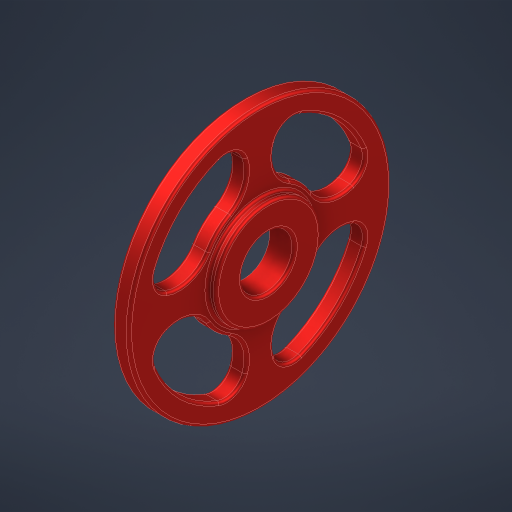
# Autodesk Inventor part: Part5
Saved by Autodesk Inventor 2024 (Build 280153000, 153)
## iProperties
Created: 2024-03-07
Part Number: Part5
Material: Aluminum, Anodized Red
Document SubType Name: Modeling
Designer: Papryk
Density: 2.7 g/cm^3
Appearance: Anodized - Red
Author: Papryk
Autodesk Inventor part; units mm, degrees
ref_plane "YZ Plane" through (0, 0, 0) normal (1, 0, 0) x (0, 1, 0)
ref_plane "XZ Plane" through (0, 0, 0) normal (0, 1, 0) x (-1, 0, 0)
ref_plane "XY Plane" through (0, 0, 0) normal (0, 0, 1) x (1, 0, 0)
sketch "Sketch1" plane through (0, 0, 0) normal (1, 0, 0) x (0, 1, 0)
  arc A0 (15.3115, -37.4941) -> (37.7556, -14.6548) centre (0, 0) ccw
  arc A1 (11.2212, -18.9232) -> (19.1161, -10.8892) centre (0, 0) ccw
  arc A2 (33.5916, -5.5323) -> (19.1161, -10.8892) centre (29.5431, -16.8287) ccw
  arc A3 (11.2212, -18.9232) -> (6.1177, -33.4899) centre (17.3418, -29.2449) ccw
  arc A4 (37.7556, -14.6548) -> (33.5916, -5.5323) centre (31.2299, -12.1219) ccw
  arc A5 (6.1177, -33.4899) -> (15.3115, -37.4941) centre (12.6651, -31.0136) ccw
  arc A6 (0, -47.5) -> (47.5, 0) centre (0, 0) ccw
  arc A7 (0, -19) -> (19, 0) centre (0, 0) ccw
  arc A8 (0, -9.5) -> (9.5, 0) centre (0, 0) ccw
  arc A9 (-37.7556, -14.6548) -> (-15.3115, -37.4941) centre (0, 0) ccw
  arc A10 (-19.1161, -10.8892) -> (-11.2212, -18.9232) centre (0, 0) ccw
  arc A11 (-19.1161, -10.8892) -> (-33.5916, -5.5323) centre (-29.5431, -16.8287) ccw
  arc A12 (-6.1177, -33.4899) -> (-11.2212, -18.9232) centre (-17.3418, -29.2449) ccw
  arc A13 (-33.5916, -5.5323) -> (-37.7556, -14.6548) centre (-31.2299, -12.1219) ccw
  arc A14 (-15.3115, -37.4941) -> (-6.1177, -33.4899) centre (-12.6651, -31.0136) ccw
  arc A15 (-47.5, 0) -> (0, -47.5) centre (0, 0) ccw
  arc A16 (-19, 0) -> (0, -19) centre (0, 0) ccw
  arc A17 (-9.5, 0) -> (0, -9.5) centre (0, 0) ccw
  arc A18 (37.7556, 14.6548) -> (15.3115, 37.4941) centre (0, 0) ccw
  arc A19 (19.1161, 10.8892) -> (11.2212, 18.9232) centre (0, 0) ccw
  arc A20 (19.1161, 10.8892) -> (33.5916, 5.5323) centre (29.5431, 16.8287) ccw
  arc A21 (6.1177, 33.4899) -> (11.2212, 18.9232) centre (17.3418, 29.2449) ccw
  arc A22 (33.5916, 5.5323) -> (37.7556, 14.6548) centre (31.2299, 12.1219) ccw
  arc A23 (15.3115, 37.4941) -> (6.1177, 33.4899) centre (12.6651, 31.0136) ccw
  arc A24 (47.5, 0) -> (0, 47.5) centre (0, 0) ccw
  arc A25 (19, 0) -> (0, 19) centre (0, 0) ccw
  arc A26 (9.5, 0) -> (0, 9.5) centre (0, 0) ccw
  arc A27 (-37.7556, 14.6548) -> (-33.5916, 5.5323) centre (-31.2299, 12.1219) ccw
  arc A28 (-33.5916, 5.5323) -> (-19.1161, 10.8892) centre (-29.5431, 16.8287) ccw
  arc A29 (-11.2212, 18.9232) -> (-19.1161, 10.8892) centre (0, 0) ccw
  arc A30 (-15.3115, 37.4941) -> (-37.7556, 14.6548) centre (0, 0) ccw
  arc A31 (-11.2212, 18.9232) -> (-6.1177, 33.4899) centre (-17.3418, 29.2449) ccw
  arc A32 (-6.1177, 33.4899) -> (-15.3115, 37.4941) centre (-12.6651, 31.0136) ccw
  arc A33 (0, 9.5) -> (-9.5, 0) centre (0, 0) ccw
  arc A34 (0, 19) -> (-19, 0) centre (0, 0) ccw
  arc A35 (0, 47.5) -> (-47.5, 0) centre (0, 0) ccw
  constraints: 72 point on circle, 36 centre point, 8 coincident, 4 tangent, 1 equal radius
extrude "Extrusion1" add sketch "Sketch1" along normal blind 6 contours A15 A35 A24 A6
extrude "Extrusion2" add sketch "Sketch1" along normal blind 9 contours A16 A34 A25 A7
fillet "Fillet1" radius 1 1 edges at (6, 47.5, 0)
fillet "Fillet2" radius 1 52 edges at (0, 47.5, 0) (9, -19, 0) (6, -19, 0) (9, 0, -9.5) (6, 9.87, 37.4314) (6, 28.8866, 28.3868) (6, 37.5979, 9.2152) (6, 25.3783, 5.5746) (6, 15.6915, 15.42) (6, 6.0167, 25.2772) (0, 9.87, 37.4314) (0, 28.8866, 28.3868) (0, 37.5979, 9.2152) (0, 25.3783, 5.5746) (0, 15.6915, 15.42) (0, 6.0167, 25.2772) (6, 15.6915, -15.42) (6, 25.3783, -5.5746) (6, 37.5979, -9.2152) (6, 28.8866, -28.3868) (6, 9.87, -37.4314) (6, 6.0167, -25.2772) (6, -9.87, -37.4314) (6, -28.8866, -28.3868) (6, -37.5979, -9.2152) (6, -25.3783, -5.5746) (6, -15.6915, -15.42) (6, -6.0167, -25.2772) (6, -37.5979, 9.2152) (6, -28.8866, 28.3868) (6, -9.87, 37.4314) (6, -6.0167, 25.2772) (6, -15.6915, 15.42) (6, -25.3783, 5.5746) (0, -37.5979, 9.2152) (0, -28.8866, 28.3868) (0, -9.87, 37.4314) (0, -6.0167, 25.2772) (0, -15.6915, 15.42) (0, -25.3783, 5.5746) (0, -37.5979, -9.2152) (0, -25.3783, -5.5746) (0, -15.6915, -15.42) (0, -6.0167, -25.2772) (0, -9.87, -37.4314) (0, -28.8866, -28.3868) (0, 6.0167, -25.2772) (0, 15.6915, -15.42) (0, 25.3783, -5.5746) (0, 37.5979, -9.2152) (0, 28.8866, -28.3868) (0, 9.87, -37.4314)
body "Solid1"
